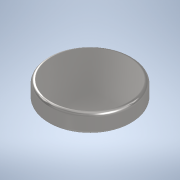
# Autodesk Inventor part: 04-02-02-020_Magnet
Saved by Autodesk Inventor 2020 (Build 240168000, 168)
## iProperties
Created: 2020-08-03
Part Number: 04-02-02-020_Magnet
Material: Edelstahl
Document SubType Name: Modeling
Designer: Eric
Density: 8 g/cm^3
Appearance: Halbpoliert
Mass: 1.86955 g
Surface Area: 3.01855 cm^2
Volume: 0.233694 cm^3
Author: Eric
Autodesk Inventor part; units mm, degrees
ref_plane "YZ Plane" through (0, 0, 0) normal (1, 0, 0) x (0, 1, 0)
ref_plane "XZ Plane" through (0, 0, 0) normal (0, 1, 0) x (-1, 0, 0)
ref_plane "XY Plane" through (0, 0, 0) normal (0, 0, 1) x (1, 0, 0)
sketch "Skizze1" plane through (0, 0, 0) normal (0, 1, 0) x (-1, 0, 0)
  circle A0 centre (0, 0) radius 6
  dimension "d1" = 12
  constraints: 1 centre point
  measures "d1" diameter of A0
extrude "Extrusion1" add sketch "Skizze1" along normal blind 2.6
fillet "Rundung1" radius 0.5 2 edges at (6, 2.6, 0) (6, 0, 0)
